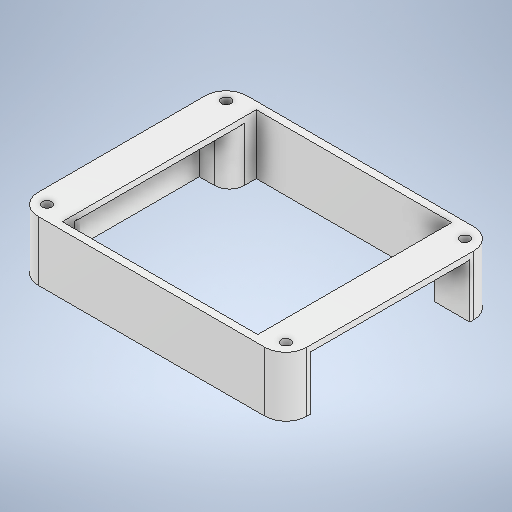
# Autodesk Inventor part: Módulo de fixação Eletrônicos
Saved by Autodesk Inventor 2025 (Build 290162000, 162)
## iProperties
Created: 2024-04-25
Part Number: Módulo de fixação Eletrônicos
Material: PPS Plastic
Document SubType Name: Modeling
Designer: kaike
Density: 1.637 g/cm^3
Appearance: Smooth - White
Mass: 31.4308 g
Surface Area: 149.197 cm^2
Volume: 19.2003 cm^3
Author: kaike
Autodesk Inventor part; units mm, degrees
ref_plane "YZ Plane" through (0, 0, 0) normal (1, 0, 0) x (0, 1, 0)
ref_plane "XZ Plane" through (0, 0, 0) normal (0, 1, 0) x (-1, 0, 0)
ref_plane "XY Plane" through (0, 0, 0) normal (0, 0, 1) x (1, 0, 0)
sketch "Sketch1" plane through (0, 0, 0) normal (0, 1, 0) x (-1, 0, 0)
  line L0 (0, 0) -> (90, 0)
  line L1 (90, 0) -> (90, -70)
  line L2 (90, -70) -> (0, -70)
  circle A0 centre (85, -65) radius 1.6095
  circle A1 centre (85, -5) radius 1.6095
  circle A2 centre (5, -65) radius 1.6095
  circle A3 centre (5, -5) radius 1.6095
  line L3 (11.9037, -61.65) -> (11.9037, -67.5)
  line L4 (11.9037, -67.5) -> (77.409, -67.5)
  line L5 (77.409, -67.5) -> (77.409, -58.5)
  line L6 (87.5, -35) -> (87.5, -58.5)
  line L7 (87.5, -58.5) -> (77.409, -58.5)
  line L8 (11.9037, -61.65) -> (0, -61.65)
  line L9 (0, -61.65) -> (0, -70)
  line L10 (11.9037, -8.35) -> (11.9037, -2.5)
  line L11 (11.9037, -2.5) -> (77.409, -2.5)
  line L12 (77.409, -2.5) -> (77.409, -11.5)
  line L13 (87.5, -35) -> (87.5, -11.5)
  line L14 (87.5, -11.5) -> (77.409, -11.5)
  line L15 (11.9037, -8.35) -> (0, -8.35)
  line L16 (0, -8.35) -> (0, 0)
  line L17 (99.038, -35) -> (-9.0118, -35) construction
  point P0 (11.9037, -5.425)
  dimension "d34" = 70
  dimension "d35" = 60
  dimension "d37" = 10.091
  dimension "d38" = 65.5053
  dimension "d39" = 60
  dimension "d40" = 70
  dimension "d41" = 9
  dimension "d43" = 90
  dimension "d44" = 11.9037
  dimension "d45" = 3.219
  dimension "d46" = 47
  dimension "d47" = 5.85
  dimension "d48" = 8.35
  dimension "d49" = 5
  dimension "d50" = 5
  dimension "d51" = 5
  dimension "d52" = 5
  constraints: 36 end point, 4 centre point, 3 horizontal, 3 perpendicular, 2 vertical, 1 midpoint, 1 parallel
  measures "d34" distance of L0.end L1.end
  measures "d35" distance of A1.centre A0.centre
  measures "d37" distance of L6.end L5.end
  measures "d38" distance from line of point (11.904, -5.425) L12
  measures "d39" distance of A3.centre A2.centre
  measures "d40" distance of L0.start L2.end
  measures "d41" distance of L4.end L5.end
  measures "d43" distance of L1.end L2.end
  measures "d44" distance of L10.start L15.end
  measures "d45" diameter of A0
  measures "d46" distance of L6.end L13.end
  measures "d47" distance of L11.start L10.start
  measures "d48" distance of L8.end L2.end
  measures "d49" distance from line of L2 A2.centre
  measures "d50" distance from line of L9 A2.centre
  measures "d51" distance from line of L1 A1.centre
  measures "d52" distance from line of L0 A1.centre
extrude "Extrusion1" add sketch "Sketch1" along normal blind 20 contours L0 L1 L2 L9 L8 L3 L4 L5 L7 L6 L13 L14 L12 L11 L10 L15 L16 | A0 | A1 | A2 | A3
sketch "Sketch2" plane through (0, 20, 0) normal (0, 1, 0) x (1, 0, 0)
  line L0 (0, 70) -> (-90, 70) projected
  circle A0 centre (-4.9798, 65) radius 1.6095
  line L1 (-90, 70) -> (-90, 0) projected
  circle A1 centre (-85.0202, 65) radius 1.6095
  circle A2 centre (-4.9798, 5) radius 1.6095
  circle A3 centre (-85.0202, 5) radius 1.6095
  point P0 (0, 0)
  constraints: 4 centre point
extrude "Extrusion2" cut sketch "Sketch2" against normal blind 30
fillet "Fillet1" radius 7 4 edges at (-90, 10, 0) (-90, 10, -70) (0, 10, -70) (0, 10, 0)
sketch "Sketch4" plane through (0, 20, 0) normal (0, 1, 0) x (1, 0, 0)
  line L0 (-77.409, 11.5) -> (-77.409, 58.5)
  line L1 (-77.409, 58.5) -> (-87.5, 58.5)
  line L2 (-87.5, 58.5) -> (-87.5, 11.5)
  line L3 (-87.5, 11.5) -> (-77.409, 11.5)
  point P0 (0, 0)
  constraints: 8 end point, 2 perpendicular, 1 vertical
extrude "Extrusion3" add sketch "Sketch4" against normal blind 2
sketch "Sketch5" plane through (0, 20, 0) normal (0, 1, 0) x (1, 0, 0)
  line L0 (-11.9037, 61.65) -> (-11.9037, 8.35)
  line L1 (-11.9037, 8.35) -> (0, 8.35)
  line L2 (0, 8.35) -> (0, 61.65)
  line L3 (0, 61.65) -> (-11.9037, 61.65)
  line L4 (-11.9037, 61.65) -> (-77.409, 61.65)
  line L5 (-77.409, 58.5) -> (-77.409, 67.5) projected
  line L6 (-77.409, 67.5) -> (-77.409, 61.65)
  line L7 (-11.9037, 61.65) -> (-11.9037, 67.5)
  line L8 (-11.9037, 67.5) -> (-77.409, 67.5)
  line L9 (-11.9037, 2.5) -> (-77.409, 2.5) projected
  line L10 (-11.9037, 8.35) -> (-11.9037, 2.5)
  line L11 (-11.9037, 2.5) -> (-77.409, 2.5)
  line L12 (-77.409, 2.5) -> (-77.409, 8.35)
  line L13 (-77.409, 8.35) -> (-11.9037, 8.35)
  point P0 (0, 0)
  constraints: 24 end point, 7 perpendicular, 3 point on line, 2 vertical, 1 collinear, 1 horizontal
extrude "Extrusion4" add sketch "Sketch5" against normal blind 2
fillet "Fillet2" radius 5 1 edges at (-77.409, 9, -58.5)
fillet "Fillet3" radius 5 1 edges at (-77.409, 9, -11.5)
fillet "Fillet4" radius 5 4 edges at (-77.409, 19, -61.65) (-11.9037, 19, -61.65) (-11.9037, 19, -8.35) (-77.409, 19, -8.35)
sketch "Sketch6" plane through (0, 20, 0) normal (0, 1, 0) x (1, 0, 0)
  line L0 (-77.409, 67.5) -> (-11.9037, 67.5)
  line L1 (-11.9037, 67.5) -> (-11.9037, 2.5)
  line L2 (-11.9037, 2.5) -> (-77.409, 2.5)
  line L3 (-77.409, 2.5) -> (-77.409, 67.5)
  point P0 (0, 0)
  constraints: 8 end point, 1 perpendicular
extrude "Extrusion5" cut sketch "Sketch6" against normal blind 10
body "Solid1"
